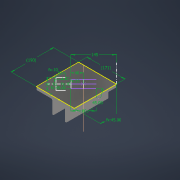
# Autodesk Inventor part: support_basePart
Saved by Autodesk Inventor 2021 (Build 250183000, 183)
## iProperties
Created: 2021-05-24
Part Number: support_basePart
Material: Steel, High Strength, Low Alloy
Document SubType Name: Modeling
Designer: Watchdog
Density: 7.85 g/cm^3
Appearance: Steel - Polished
Author: Watchdog
Autodesk Inventor part; units mm, degrees
ref_plane "YZ Plane" through (0, 0, 0) normal (1, 0, 0) x (0, 1, 0)
ref_plane "XZ Plane" through (0, 0, 0) normal (0, 1, 0) x (-1, 0, 0)
ref_plane "XY Plane" through (0, 0, 0) normal (0, 0, 1) x (1, 0, 0)
sketch "Sketch1" plane through (0, 0, 0) normal (0, 0, 1) x (1, 0, 0)
  line L0 (-33, 0) -> (33, 0)
  line L1 (33, 0) -> (33, -58)
  line L2 (33, -58) -> (-33, -58)
  line L3 (-33, -58) -> (-33, 0)
  point P0 (0, 0)
  dimension "d0" = 58
  dimension "d1" = 66
  dimension "d2" = 33
  dimension "d3" = 0
  constraints: 8 end point, 2 parallel, 1 horizontal, 1 perpendicular
  measures "d0" distance of L2.end L0.start
  measures "d1" distance of L0.start L0.end
  measures "d2" distance from line of point (0, 0) L3
  measures "d3" distance from line of point (0, 0) L0
extrude "clamp_base" add sketch "Sketch1" against normal blind 190
sketch "Sketch2" plane through (0, 0, 0) normal (0, 0, 1) x (1, 0, 0)
  line L0 (-25, -58) -> (25, -58)
  line L1 (25, -58) -> (25, -8)
  line L2 (25, -8) -> (-25, -8)
  line L3 (-25, -8) -> (-25, -58)
  line L4 (-33, -58) -> (33, -58) projected
  point P0 (0, 0)
  dimension "d6" = 50
  dimension "d7" = 50
  dimension "d8" = 25
  constraints: 8 end point, 2 parallel, 1 collinear, 1 horizontal, 1 perpendicular
  measures "d6" distance between parallel lines of L1 L3
  measures "d7" distance of L2.end L0.start
  measures "d8" distance from line of point (0, 0) L3
extrude "clamp_extrusion" cut sketch "Sketch2" against normal through all
sketch "Sketch4" plane through (-33, 0, 0) normal (0, 1, 0) x (1, 0, 0)
  line L0 (-70, 190) -> (101, 190)
  line L1 (101, 190) -> (101, 0)
  line L2 (101, 0) -> (-70, 0)
  line L3 (-70, 0) -> (-70, 190)
  line L4 (66, 0) -> (0, 0) projected
  line L5 (0, 190) -> (66, 190) projected
  line L6 (0, 0) -> (0, 190) projected
  line L7 (66, 0) -> (66, 190) projected
  point P0 (33, 0)
  dimension "d35" = 0
  dimension "d36" = 0
  dimension "d37" = 70
  dimension "d38" = 35
  constraints: 8 end point, 2 parallel, 1 horizontal, 1 perpendicular
  measures "d35" distance between parallel lines of L2 L4
  measures "d36" distance between parallel lines of L0 L5
  measures "d37" distance between parallel lines of L6 L3
  measures "d38" distance between parallel lines of L1 L7
extrude "platform" add sketch "Sketch4" along normal blind 15
sketch "Sketch8" plane through (33, -58, 0) normal (1, 0, 0) x (0, 0, -1)
  line L0 (0, 0) -> (0, 58) projected
  line L1 (190, 58) -> (190, 0) projected
  point P0 (45, 24.0271)
  point P1 (145, 24.0271)
  dimension "d51" = 45
  dimension "d60" = 100
  dimension "d61" = 190
  measures "d51" distance from line of L0 point (45, 24.027)
  measures "d60" distance of point (145, 24.027) point (45, 24.027)
  measures "d61" distance between parallel lines of L1 L0
hole "clampHole" at (33, -33.9729, -45) at (33, -33.9729, -145) direction (-1, 0, 0) diameter 10 end through all
sketch "tabWeld" plane through (-33, 15, 0) normal (0, 1, 0) x (1, 0, 0)
  line L0 (16.5007, 69.4383) -> (73.0693, 126.0068)
  line L1 (-19.5617, 105.5007) -> (37.0068, 162.0693)
  line L2 (-70, 0) -> (101, 0) projected
  line L3 (-70, 190) -> (-70, 0) projected
  line L4 (16.5007, 69.4383) -> (-19.5617, 105.5007)
  line L5 (-1.5305, 87.4695) -> (55.0381, 144.0381)
  line L6 (101, 0) -> (101, 190) projected
  line L7 (8.7226, 133.785) -> (44.785, 97.7226)
  line L8 (101, 190) -> (-70, 190) projected
  line L9 (101, 190) -> (17.4246, 273.5754)
  point P0 (33, 0)
  point P1 (26.7538, 115.7538)
  dimension "d63" = 80
  dimension "d64" = 51
  dimension "d67" = 45
  dimension "d68" = 171
  dimension "d70" = 40
  dimension "d71" = 190
  dimension "d88" = 45
  dimension "d89" = 145
  constraints: 13 end point, 5 midpoint, 4 parallel, 2 perpendicular
  measures "d63" distance of L0.start L0.end
  measures "d64" distance between parallel lines of L1 L0
  measures "d67" angle of L2 L0
  measures "d68" distance between parallel lines of L6 L3
  measures "d70" distance from line of L4 point (26.754, 115.754)
  measures "d71" distance between parallel lines of L2 L8
  measures "d88" angle of L2 L9
  measures "d89" distance from line of L9.end L4
ref_plane "Work Plane4" through (-24.2774, 15, -133.785) normal (-0.7071068, 0, 0.7071068) x (0.7071068, 0, 0.7071068)
sketch "reelWeld" plane through (-33, 15, 0) normal (0, 1, 0) x (1, 0, 0)
  line L0 (-38.7868, 99.7107) -> (-60, 78.4975)
  line L1 (-70, 0) -> (101, 0) projected
  line L2 (-10.5025, 29) -> (10.7107, 50.2132)
  line L3 (-70, 190) -> (-70, 0) projected
  line L4 (-1.5305, 87.4695) -> (55.0381, 144.0381) projected
  line L5 (-1.5305, 87.4695) -> (-54.9116, 34.0884)
  line L6 (-60, 78.4975) -> (-10.5025, 29)
  point P0 (33, 0)
  dimension "d75" = 45
  dimension "d77" = 30
  dimension "d78" = 70
  dimension "d79" = 70
  dimension "d86" = 35
  dimension "d87" = 10
  constraints: 8 end point, 1 collinear, 1 parallel
  measures "d75" angle of L1 L0
  measures "d77" distance of L0.start L0.end
  measures "d78" distance between parallel lines of L2 L0
  measures "d79" distance of L2.end L0.start
  measures "d86" distance from line of L4.start L0
  measures "d87" distance from line of L3 L0.end
fillet "Fillet1" radius 2 2 edges at (33, 0, -95) (-33, 0, -95)
chamfer "Chamfer1" distance 2 angle 45 28 edges at (68, 15, -95) (-17.5, 15, -190) (-103, 15, -95) (-17.5, 15, 0) (51.5, 0, -190) (33.5858, -0.5858, -190) (33, -30, -190) (68, 0, -95) (51.5, 0, 0) (33.5858, -0.5858, 0) (33, -30, 0) (-33, -30, -190) (-33.5858, -0.5858, -190) (-69, 0, -190) (-103, 0, -95) (-69, 0, 0) (-33.5858, -0.5858, 0) (-33, -30, 0) (68, 7.5, -190) (-103, 7.5, -190) (-103, 7.5, 0) (68, 7.5, 0) (0, -8, -190) (25, -33, -190) (-25, -33, -190) (0, -8, 0) (-25, -33, 0) (25, -33, 0)
equation "\"d0\" = support_frame_squareBarDimension + support_baseClamp_thickness"
equation "\"d1\" = support_frame_squareBarDimension + 2 * support_baseClamp_thickness"
equation "\"d2\" = 0.5 * d1"
equation "\"d4\" = width"
equation "\"d6\" = support_frame_squareBarDimension"
equation "\"d7\" = support_frame_squareBarDimension"
equation "\"d8\" = 0.5 * d6"
equation "\"d37\" = 2 * support_baseClamp_platformLengthBuffer"
equation "\"d38\" = support_baseClamp_platformLengthBuffer"
equation "\"d13\" = support_baseClamp_platformThickness"
equation "\"d51\" = -0.5 * d60 + 0.5 * d61"
equation "\"d60\" = clampHoleSpacing"
equation "\"d53\" = clampHoleDiameter"
equation "\"d75\" = d67"
equation "\"d79\" = d78"
equation "\"hoop_width_large\" = 51"
equation "\"width\" = clampHoleDiameter + clampHoleSpacing + 2 * buffer"
equation "\"clampHoleSpacing\" = support_frame_clampHoleSpacing"
equation "\"clampHoleDiameter\" = support_frame_clampHoleDiameter"
equation "\"d12\" = -y + r - d15"
equation "\"d15\" = hoop_width_large"
equation "\"sleeveHoleDiameter\" = support_baseClamp_sleeveHoleDiameter"
equation "\"theta\" = hoop_angle_z"
equation "\"phi\" = support_baseClamp_sleeveSweepTerminationAngle"
equation "\"support_frame_squareBarDimension\" = 50"
equation "\"support_baseClamp_thickness\" = 8"
equation "\"support_baseClamp_sleeveHoleDiameter\" = 12"
equation "\"hoop_angle_z\" = 45deg"
equation "\"support_baseClamp_sleeveSweepTerminationAngle\" = 55deg"
equation "\"support_baseClamp_platformThickness\" = 15"
equation "\"support_baseClamp_platformWidthBuffer\" = 0"
equation "\"support_baseClamp_platformLengthBuffer\" = 35"
equation "\"rack_tooth_thickness\" = 5"
equation "\"rack_tooth_addendum\" = 5"
equation "\"rack_tooth_dedendum\" = 5"
equation "\"hoop_thickness_large\" = 4"
equation "\"hoop_width_medium\" = 33.7"
equation "\"hoop_thickness_medium\" = 3.2"
equation "\"hoop_width_small\" = 25.4"
equation "\"hoop_thickness_small\" = 2"
equation "\"hoop_bearing_length\" = 5deg"
equation "\"hoop_cable_diam\" = 5"
equation "\"hoop_cable_pulley_diam\" = 22"
equation "\"secure_arm_radii\" = 9"
equation "\"secure_arm_angle\" = 35deg"
equation "\"support_frame_endHoleBuffer\" = 25"
equation "\"hoop_tabs_thickness\" = 6"
equation "\"support_frame_squareBarThickness\" = 5"
equation "\"wheelchair_deployed_length\" = 1067"
equation "\"wheelchair_deployed_height\" = 914"
equation "\"hoop_tabs_hole\" = 12"
equation "\"wheelchair_deployed_width\" = 635"
equation "\"support_frame_squareBarFillet\" = 2"
equation "\"sm_varx_pinPlate_thickness\" = 5"
equation "\"sm_varx_member_tolerance\" = 0.5"
equation "\"sm_varx_pinPlate_holeDiameter\" = 5"
equation "\"sm_varx_squareBarThickness\" = 2.5"
equation "\"hoop_bushing23_radialInterference\" = 0"
equation "\"hoop_bushing12_radialInterference\" = 0"
equation "\"hoop_bushing12_od\" = -2 * hoop_thickness_large + hoop_width_large + hoop_bushing12_radialInterference"
equation "\"buffer\" = 40"
equation "\"support_frame_clampHoleSpacing\" = 100"
equation "\"support_frame_clampHoleDiameter\" = 10"
equation "\"y\" = 450"
equation "\"r\" = 1650"
body "Solid1"
